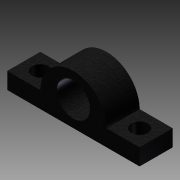
# Autodesk Inventor part: axle bearing
Saved by Autodesk Inventor 2011 (Build 150239000, 239)
## iProperties
Created: 2013-01-17
Part Number: axle bearing
Document SubType Name: Modeling
Designer: Christopher
Density: 1 g/cm^3
Author: Christopher
Autodesk Inventor part; units mm, degrees
ref_plane "YZ Plane" through (0, 0, 0) normal (1, 0, 0) x (0, 1, 0)
ref_plane "XZ Plane" through (0, 0, 0) normal (0, 1, 0) x (-1, 0, 0)
ref_plane "XY Plane" through (0, 0, 0) normal (0, 0, 1) x (1, 0, 0)
sketch "Sketch1" plane through (0, 0, 0) normal (0, 0, 1) x (1, 0, 0)
  line L0 (0, 0) -> (50.8, 0)
  line L1 (50.8, 0) -> (50.8, 6.35)
  line L2 (0, 6.35) -> (0, 0)
  arc A0 (38.1, 6.35) -> (12.7, 6.35) centre (25.4, 6.35) ccw
  line L3 (25.4, 6.35) -> (38.1, 6.35) construction
  line L4 (25.4, 6.35) -> (12.7, 6.35) construction
  line L5 (12.7, 6.35) -> (0, 6.35)
  line L6 (38.1, 6.35) -> (50.8, 6.35)
  circle A1 centre (25.4, 9.525) radius 6.35
  point P0 (25.4, 0)
  dimension "d0" = 50.8
  dimension "d2" = 12.7
  dimension "d3" = 180
  dimension "d4" = 6.35
  dimension "d5" = 12.7
  dimension "d6" = 9.525
  constraints: 14 end point, 3 equal length, 2 centre point, 2 point on circle, 1 horizontal, 1 horizontal alignment, 1 midpoint, 1 perpendicular, 1 vertical alignment
  measures "d0" distance of L2.start L1.end
  measures "d2" radius of A0
  measures "d3" angle of L3 L4
  measures "d4" distance of L0.end L1.end
  measures "d5" diameter of A1
  measures "d6" distance from line of L0 A1.centre
extrude "Extrusion1" add sketch "Sketch1" against normal blind 12.7
sketch "Sketch2" plane through (0, 6.35, 0) normal (0, 1, 0) x (1, 0, 0)
  line L0 (0, 0) -> (0, 12.7) projected
  line L1 (50.8, 0) -> (50.8, 12.7) projected
  point P0 (6.35, 6.35)
  point P1 (44.45, 6.35)
  dimension "d9" = 6.35
  dimension "d10" = 6.35
  measures "d9" distance from line of L1 point (44.45, 6.35)
  measures "d10" distance from line of L0 point (6.35, 6.35)
hole "Hole1" at (6.35, 6.35, -6.35) at (44.45, 6.35, -6.35) direction (0, -1, 0) diameter 6.35 depth 25.4 tip angle 118
body "Solid1"
